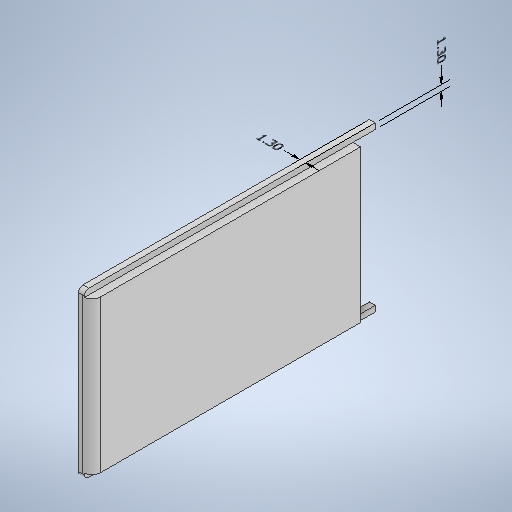
# Autodesk Inventor part: upper cover
Saved by Autodesk Inventor 2025.4 (Build 294407000, 407)
## iProperties
Created: 2026-03-11
Part Number: upper cover
Material: Generic
Document SubType Name: Modeling
Designer: Amir
Density: 1 g/cm^3
Appearance: Default
Author: Amir
## iProperties of the stored document upper cover_3DPrint.ipt
Created: 2026-04-12
Part Number: upper cover_3DPrint
Material: Generic
Document SubType Name: Modeling
Designer: Amir
Density: 1 g/cm^3
Appearance: Default
Author: Amir
Autodesk Inventor part; units mm, degrees
ref_plane "YZ Plane" through (0, 0, 0) normal (1, 0, 0) x (0, 1, 0)
ref_plane "XZ Plane" through (0, 0, 0) normal (0, 1, 0) x (-1, 0, 0)
ref_plane "XY Plane" through (0, 0, 0) normal (0, 0, 1) x (1, 0, 0)
sketch "Sketch1" plane through (0, 0, 0) normal (0, 0, 1) x (1, 0, 0)
  line L0 (13.5206, 26.4904) -> (14.8206, 26.4904)
  line L1 (14.8206, 26.4904) -> (14.8206, 25.1904)
  line L2 (14.8206, 25.1904) -> (16.5206, 25.1904)
  line L3 (16.5206, -8.8096) -> (14.8206, -8.8096)
  line L4 (14.8206, -8.8096) -> (14.8206, -10.1096)
  line L5 (14.8206, -10.1096) -> (13.5206, -10.1096)
  line L6 (16.5206, 25.1904) -> (16.5206, -8.8096)
  line L7 (13.5206, 25.1904) -> (14.8206, 25.1904)
  line L8 (14.8206, -8.8096) -> (13.5206, -8.8096)
  line L9 (13.5206, 26.4904) -> (13.5206, -10.1096)
  dimension "d2" = 1.3
  dimension "d15" = 3
  dimension "d16" = 1.3
  dimension "d17" = 1.3
  dimension "d18" = 1.3
  dimension "d19" = 34
  dimension "d20" = 36.6
  dimension "d21" = 1.7
  constraints: 20 end point, 4 point on line, 3 parallel, 2 vertical, 1 horizontal, 1 perpendicular
  measures "d2" distance of L0.start L0.end
  measures "d15" distance between parallel lines of L9 L6
  measures "d16" distance of L5.start L5.end
  measures "d17" distance of L4.start L5.start
  measures "d18" distance of L0.end L1.end
  measures "d19" distance between parallel lines of L3 L2
  measures "d20" distance of L0.start L5.end
  measures "d21" distance of L1.end L2.end
extrude "Extrusion1" add sketch "Sketch1" along normal blind 60
extrude "Extrusion2" add sketch "Sketch1" against normal blind 5 contours L0 L1 L7 L9 | L8 L4 L5 L9
fillet "Fillet2" radius 1 2 edges at (14.1706, 26.4904, 60) (14.1706, -10.1096, 60)
fillet "Fillet3" radius 2 1 edges at (16.5206, 8.1904, 60)
body "Solid1"
